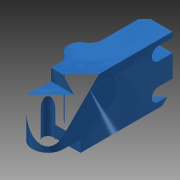
# Autodesk Inventor part: OfflineBowdenExtruderIdler
Saved by Autodesk Inventor 2015 SP1 (Build 190203100, 203)
## iProperties
Created: 2015-04-29
Part Number: OfflineBowdenExtruderIdler
Material: Generic
Document SubType Name: Modeling
Designer: Jack
Density: 1 g/cm^3
Appearance: Cyan
Author: Jack
Autodesk Inventor part; units mm, degrees
ref_plane "YZ Plane" through (0, 0, 0) normal (1, 0, 0) x (0, 1, 0)
ref_plane "XZ Plane" through (0, 0, 0) normal (0, 1, 0) x (-1, 0, 0)
ref_plane "XY Plane" through (0, 0, 0) normal (0, 0, 1) x (1, 0, 0)
sketch "Sketch1" plane through (0, 0, 0) normal (0, 0, 1) x (1, 0, 0)
  arc A0 (-4.75, 2.2361) -> (5.25, 0) centre (0, 0) ccw
  line L0 (5.25, 0) -> (5.25, 37)
  line L1 (5.25, 37) -> (-4.25, 37)
  arc A1 (-4.25, 19.4922) -> (-4.75, 11.5078) centre (-4.5, 15.5) ccw
  line L2 (-4.25, 37) -> (-4.25, 19.4922)
  line L3 (-4.75, 11.5078) -> (-4.75, 2.2361)
  dimension "d0" = 10.5
  dimension "d1" = 37
  dimension "d3" = 4.5
  dimension "d4" = 15.5
  dimension "d5" = 8
  dimension "d22" = 10
  dimension "d23" = 9.5
  constraints: 8 end point, 4 point on circle, 2 centre point, 2 vertical, 1 coincident, 1 perpendicular, 1 tangent
  measures "d0" diameter of A0
  measures "d1" distance from line of point (0, 0) L1
  measures "d3" horizontal distance of point (0, 0) A1.centre
  measures "d4" vertical distance of point (0, 0) A1.centre
  measures "d5" diameter of A1
  measures "d22" distance between parallel lines of L0 L3
  measures "d23" distance between parallel lines of L0 L2
extrude "Extrusion1" add sketch "Sketch1" along normal blind 20
sketch "Sketch2" plane through (0, 0, 20) normal (0, 0, 1) x (1, 0, 0)
  arc A0 (-4.75, 2.2361) -> (5.25, 0) centre (0, 0) ccw projected
  line L0 (5.25, 0) -> (5.25, 37) projected
  line L1 (-4.75, 11.5078) -> (-4.75, 2.2361) projected
  line L2 (-4.75, 5.8) -> (5.25, 5.8)
  dimension "d9" = 5.8
  constraints: 2 end point, 2 point on line, 1 perpendicular
  measures "d9" distance from line of A0.centre L2
extrude "Extrusion2" cut sketch "Sketch2" against normal blind 4
sketch "Sketch3" plane through (0, 0, 0) normal (0, 0, -1) x (-1, 0, 0)
  arc A0 (-5.25, 0) -> (4.75, 2.2361) centre (0, 0) ccw projected
  line L0 (4.75, 2.2361) -> (4.75, 11.5078) projected
  line L1 (-5.25, 37) -> (-5.25, 0) projected
  line L2 (4.75, 5.8) -> (-5.25, 5.8) projected
extrude "Extrusion3" cut sketch "Sketch3" against normal blind 4
fillet "Fillet1" radius 4 2 edges at (-4.25, 19.4922, 10) (-4.75, 11.5078, 10)
sketch "Sketch4" plane through (0, 0, 16) normal (0, 0, 1) x (1, 0, 0)
  arc A0 (-4.75, 2.2361) -> (5.25, 0) centre (0, 0) ccw projected
hole "Hole1" at (0, 0, 16) direction (0, 0, -1) diameter 3.5 end through all
sketch "Sketch5" plane through (5.25, 37, 20) normal (1, 0, 0) x (0, 0, -1)
  line L0 (20, 0) -> (20, -31.2) projected
  line L1 (20, 0) -> (0, 0) projected
  arc A0 (1.75, -4.8) -> (6.25, -4.8) centre (4, -4.8) ccw
  arc A1 (13.75, -4.8) -> (18.25, -4.8) centre (16, -4.8) ccw
  line L2 (6.25, -4.8) -> (6.25, 0)
  line L3 (1.75, -4.8) -> (1.75, 0)
  line L4 (13.75, -4.8) -> (13.75, 0)
  line L5 (18.25, -4.8) -> (18.25, 0)
  point P0 (20, -37)
  dimension "d24" = 4.5
  dimension "d25" = 4.8
  dimension "d26" = 12
  dimension "d27" = 4
  constraints: 8 end point, 4 perpendicular, 4 point on circle, 4 point on line, 4 tangent, 2 centre point, 1 equal radius, 1 horizontal alignment
  measures "d24" diameter of A0
  measures "d25" distance from line of L1 A0.centre
  measures "d26" distance of A1.centre A0.centre
  measures "d27" distance from line of L0 A1.centre
extrude "Extrusion4" cut sketch "Sketch5" against normal up to next
chamfer "Chamfer1" distance 2 angle 45 3 edges at (-4.25, 37, 19.125) (-4.25, 37, 10) (-4.25, 37, 0.875)
body "Solid1"
